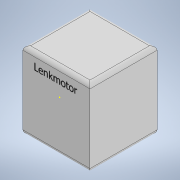
# Autodesk Inventor part: Lenkmotor
Saved by Autodesk Inventor 2021 (Build 250183000, 183)
## iProperties
Created: 2021-01-25
Part Number: Lenkmotor
Material: Generisch
Document SubType Name: Modeling
Designer: casa2
Density: 1 g/cm^3
Appearance: Vorgabe
Author: casa2
Autodesk Inventor part; units mm, degrees
ref_plane "YZ Plane" through (0, 0, 0) normal (1, 0, 0) x (0, 1, 0)
ref_plane "XZ Plane" through (0, 0, 0) normal (0, 1, 0) x (-1, 0, 0)
ref_plane "XY Plane" through (0, 0, 0) normal (0, 0, 1) x (1, 0, 0)
sketch "Skizze1" plane through (0, 0, 0) normal (0, 0, 1) x (1, 0, 0)
  line L0 (-19.1926, 13.6827) -> (15.8074, 13.6827)
  line L1 (15.8074, 13.6827) -> (15.8074, -26.3173)
  line L2 (15.8074, -26.3173) -> (-19.1926, -26.3173)
  line L3 (-19.1926, -26.3173) -> (-19.1926, 13.6827)
  point P0 (0, 0)
  dimension "d0" = 35
  dimension "d1" = 40
  constraints: 8 end point, 2 parallel, 1 horizontal, 1 perpendicular
  measures "d0" distance of L0.start L0.end
  measures "d1" distance of L0.end L1.end
extrude "Extrusion1" add sketch "Skizze1" along normal blind 35
fillet "Rundung1" radius 2 8 edges at (-19.1926, 13.6827, 17.5) (15.8074, 13.6827, 17.5) (-1.6926, 13.6827, 35) (-1.6926, 13.6827, 0) (-1.6926, -26.3173, 0) (-19.1926, -26.3173, 17.5) (15.8074, -26.3173, 17.5) (-1.6926, -26.3173, 35)
sketch "Skizze2" plane through (0, 0, 35) normal (0, 0, 1) x (1, 0, 0)
  line L0 (-13.5333, 9.2381) -> (11.0513, 9.2381) construction
  line L1 (11.0513, 9.2381) -> (11.0513, -21.0985) construction
  line L2 (11.0513, -21.0985) -> (-13.5333, -21.0985) construction
  line L3 (-13.5333, -21.0985) -> (-13.5333, 9.2381) construction
  point P0 (0, 0)
  constraints: 2 other
